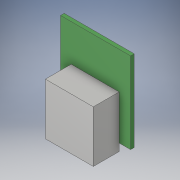
# Autodesk Inventor part: Battery-Management
Saved by Autodesk Inventor 2019 (Build 230136000, 136)
## iProperties
Created: 2018-11-25
Part Number: Battery-Management
Material: Generic
Document SubType Name: Modeling
Designer: lateSWE
Density: 1 g/cm^3
Appearance: Default
Author: lateSWE
Autodesk Inventor part; units mm, degrees
ref_plane "YZ Plane" through (0, 0, 0) normal (1, 0, 0) x (0, 1, 0)
ref_plane "XZ Plane" through (0, 0, 0) normal (0, 1, 0) x (-1, 0, 0)
ref_plane "XY Plane" through (0, 0, 0) normal (0, 0, 1) x (1, 0, 0)
sketch "Sketch1" plane through (0, 0, 0) normal (0, 0, 1) x (1, 0, 0)
  line L0 (0, 0) -> (19, 0)
  line L1 (19, 0) -> (19, 22)
  line L2 (19, 22) -> (0, 22)
  line L3 (0, 22) -> (0, 0)
  dimension "d0" = 19
  dimension "d1" = 22
  constraints: 8 end point, 2 parallel, 1 horizontal, 1 perpendicular
  measures "d0" distance of L2.end L1.end
  measures "d1" distance of L1.end L0.end
extrude "Extrusion1" add sketch "Sketch1" along normal blind 1
sketch "Sketch2" plane through (0, 0, 1) normal (0, 0, 1) x (1, 0, 0)
  line L0 (0, 0) -> (19, 0) projected
  line L1 (0, 0) -> (2.9, 0)
  line L2 (2.9, 0) -> (2.9, 12)
  line L3 (2.9, 12) -> (0, 12)
  line L4 (0, 12) -> (0, 0)
  line L5 (2.9, 12) -> (15.9, 12)
  line L6 (15.9, 12) -> (15.9, -2)
  line L7 (15.9, -2) -> (2.9, -2)
  line L8 (2.9, -2) -> (2.9, 12)
  dimension "d4" = 2.9
  dimension "d5" = 12
  dimension "d6" = 13
  dimension "d7" = 14
  constraints: 16 end point, 4 parallel, 2 horizontal, 2 perpendicular
  measures "d4" distance of L3.end L2.end
  measures "d5" distance of L2.end L1.end
  measures "d6" distance of L6.end L7.end
  measures "d7" distance of L5.end L6.end
extrude "Extrusion2" add sketch "Sketch2" along normal blind 7 contours L2 L5 L6 L0 | L0 L6 L7 L8
sketch "Sketch3" plane through (0, 0, 0) normal (0, 0, -1) x (-1, 0, 0)
  line L0 (-19, 0) -> (-19, 22) projected
  line L1 (-19, 0) -> (-14, 0)
  line L2 (-14, 0) -> (-14, 5)
  line L3 (-14, 5) -> (-19, 5)
  line L4 (-19, 5) -> (-19, 0)
  line L5 (-14, 0) -> (-6, 0)
  line L6 (-6, 0) -> (-6, 5.5)
  line L7 (-6, 5.5) -> (-14, 5.5)
  line L8 (-14, 5.5) -> (-14, 0)
  line L9 (-14, 0) -> (-6, 0)
  line L10 (-6, 0) -> (-6, -1.5)
  line L11 (-6, -1.5) -> (-14, -1.5)
  line L12 (-14, -1.5) -> (-14, 0)
  point P0 (0, 0)
  dimension "d10" = 5
  dimension "d11" = 5
  dimension "d12" = 8
  dimension "d13" = 5.5
  dimension "d16" = 8
  dimension "d17" = 1.5
  constraints: 24 end point, 6 parallel, 3 horizontal, 3 perpendicular
  measures "d10" distance of L3.end L2.end
  measures "d11" distance of L2.end L1.end
  measures "d12" distance of L7.end L6.end
  measures "d13" distance of L6.end L5.end
  measures "d16" distance of L10.end L11.end
  measures "d17" distance of L9.end L10.end
extrude "Extrusion3" add sketch "Sketch3" along normal blind 3 contours L2 L8 L7 L6 L5 | L5 L10 L11 L12
body "Solid1"
